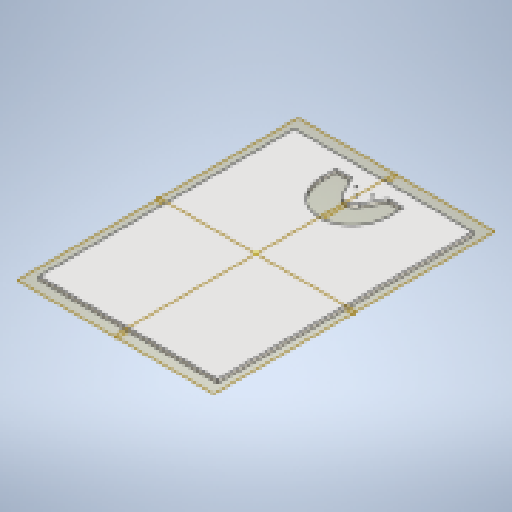
# Autodesk Inventor part: Передняя_фанера
Saved by Autodesk Inventor 2023 (Build 270158000, 158)
## iProperties
Created: 2025-10-07
Part Number: Передняя_фанера
Material: Типовые
Document SubType Name: Modeling
Designer: Олег Коноваленко
Density: 1 g/cm^3
Appearance: По умолчанию
Author: Олег Коноваленко
Autodesk Inventor part; units mm, degrees
sketch "Эскиз2" plane through (0, 0, 0) normal (0, 1, 0) x (-1, 0, 0)
  line L0 (105, 150) -> (-105, 150)
  line L1 (-105, 150) -> (-105, -150)
  line L2 (-105, -150) -> (105, -150)
  line L3 (105, -150) -> (105, 150)
  line L4 (105, 150) -> (-105, -150) construction
  line L5 (-105, 150) -> (105, -150) construction
  point P0 (0, 0)
  dimension "d0" = 300
  dimension "d1" = 210
  constraints: 12 end point, 2 midpoint, 2 parallel, 1 horizontal, 1 perpendicular
  measures "d0" distance of L0.end L1.end
  measures "d1" distance of L1.end L2.end
extrude "Выдавливание1" add sketch "Эскиз2" along normal mid plane 4
sketch "Эскиз4" plane through (0, 2, 0) normal (0, 1, 0) x (1, 0, 0)
  point P0 (0, 0)
sketch "Эскиз5" plane through (0, -2, 0) normal (0, -1, 0) x (1, 0, 0)
  line L0 (46.7, -140) -> (-46.7, -140) projected
  line L1 (-46.7, -140) -> (-46.7, -121.5234) projected
  arc A0 (-46.594, -118.6405) -> (-46.7, -121.5234) centre (-7.4334, -121.5237) ccw projected
  ellipse E0 centre (-51.6674, -118.2652) end of major axis (-52.1006, -124.2245) minor radius 5.0873 (-46.594, -118.6405) -> (-46.5935, -117.6187) ccw projected
  ellipse E1 centre (-32.0119, -116.0476) end of major axis (-31.7353, -98.7858) minor radius 14.6347 (-46.6171, -115.0294) -> (-46.5935, -117.6187) ccw projected
  spline S0 degree 3 poles (-46.6171, -115.0294) (-46.5015, -112.9122) (-46.0285, -108.6931) (-44.8405, -103.5371) (-43.2174, -98.5282) (-41.5773, -94.6618) (-39.1217, -90.0608) (-36.8431, -86.5874) (-33.6324, -82.5567) (-30.7879, -79.6008) (-26.9267, -76.2879) (-23.6107, -73.9602) (-19.2299, -71.4921) (-15.5575, -69.8842) (-10.8129, -68.3603) (-6.9178, -67.5387) (-1.9855, -67.0233) (1.9855, -67.0233) (6.9178, -67.5387) (10.8129, -68.3603) (15.5575, -69.8842) (19.2299, -71.4921) (23.6107, -73.9602) (26.9267, -76.2879) (30.7879, -79.6008) (33.6324, -82.5567) (36.8431, -86.5874) (39.1217, -90.0608) (41.5773, -94.6618) (43.2174, -98.5282) (44.8405, -103.5371) (46.0285, -108.6931) (46.5015, -112.9122) (46.6171, -115.0294) knots 1.630961 1.630961 1.630961 1.630961 1.756847 1.882733 1.945676 2.071562 2.134505 2.260391 2.323334 2.44922 2.512163 2.638049 2.700992 2.826878 2.889821 3.015707 3.07865 3.204536 3.267479 3.393365 3.456308 3.582194 3.645137 3.771023 3.833966 3.959852 4.022795 4.148681 4.211624 4.33751 4.400453 4.526339 4.652225 4.652225 4.652225 4.652225 projected
  ellipse E2 centre (32.0119, -116.0476) end of major axis (31.7353, -98.7858) minor radius 14.6347 (46.5935, -117.6187) -> (46.6171, -115.0294) ccw projected
  ellipse E3 centre (51.6674, -118.2652) end of major axis (52.1006, -124.2245) minor radius 5.0873 (46.5935, -117.6187) -> (46.594, -118.6405) ccw projected
  arc A1 (46.7, -121.5234) -> (46.594, -118.6405) centre (7.4334, -121.5237) ccw projected
  line L2 (46.7, -121.5234) -> (46.7, -140) projected
  line L3 (38.7, -118.0685) -> (38.7, -133.5234) projected
  ellipse E4 centre (0, -118.0685) end of major axis (0, -75.3678) minor radius 38.7 (38.7, -118.0685) -> (-38.7, -118.0685) ccw projected
  line L4 (-38.7, -133.5234) -> (-38.7, -118.0685) projected
  line L5 (-21.135, -133.5234) -> (-38.7, -133.5234) projected
  circle A2 centre (9.4549, -127.5234) radius 2.1 projected
  circle A3 centre (0, -118.0685) radius 2.1 projected
  circle A4 centre (-9.4549, -127.5234) radius 2.1 projected
  circle A5 centre (9.4549, -127.5234) radius 1.5
  circle A6 centre (-9.4549, -127.5234) radius 1.5
  circle A7 centre (0, -118.0685) radius 1.5
  line L6 (39.7, -118.0685) -> (39.7, -134.4459)
  line L7 (-39.7, -133.5234) -> (-39.7, -118.0685)
  line L8 (38.7, -133.5234) -> (39.7, -133.5234)
  line L9 (-38.7, -133.5234) -> (-39.7, -133.5234)
  line L10 (38.7, -133.5234) -> (21.135, -133.5234) projected
  line L11 (9.7861, -111.8345) -> (21.135, -133.5234) projected
  ellipse E5 centre (0, -118.0685) end of major axis (0, -105.6004) minor radius 11.3 (9.7861, -111.8345) -> (-9.7861, -111.8345) ccw projected
  line L12 (-21.135, -133.5234) -> (-9.7861, -111.8345) projected
  spline S1 degree 5 poles (-39.7, -118.0685) (-39.7, -116.2442) (-39.6135, -114.4198) (-39.4406, -112.6008) (-38.359, -105.0548) (-35.7799, -97.7978) (-32.9708, -92.6223) (-25.8915, -83.6065) (-16.2115, -77.5088) (-10.9886, -75.4127) (0, -73.3231) (10.9886, -75.4127) (16.2115, -77.5088) (25.8915, -83.6065) (32.9708, -92.6223) (35.7799, -97.7978) (38.359, -105.0548) (39.4406, -112.6008) (39.6135, -114.4198) (39.7, -116.2442) (39.7, -118.0685) knots 0 0 0 0 0 0 0.069589 0.069589 0.069589 0.290442 0.290442 0.290442 0.5 0.5 0.5 0.709558 0.709558 0.709558 0.930411 0.930411 0.930411 1 1 1 1 1 1
  point P0 (0, 0)
  dimension "d18" = 1
  dimension "d15" = 3
  dimension "d16" = 3
  dimension "d17" = 3
  constraints: 8 end point, 3 centre point, 3 coincident, 3 point on line, 1 horizontal alignment, 1 parallel, 1 perpendicular, 1 vertical, 8 other
  measures "d15" diameter of A5
  measures "d16" diameter of A6
  measures "d17" diameter of A7
extrude "Выдавливание3" cut sketch "Эскиз5" against normal blind 10 contours E4 L4 L9 L7 S1 L6 L8 L3 | L3 L10 L11 E5 L12 L5 L4 E4 | A5 | A6 | A7
